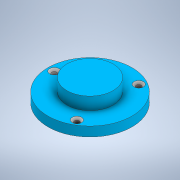
# Autodesk Inventor part: EChem _S200 Cap Base
Saved by Autodesk Inventor 2021 (Build 250183000, 183)
## iProperties
Created: 2020-07-06
Part Number: EChem _S200 Cap Base
Material: Generic
Document SubType Name: Modeling
Designer: jgray
Density: 1 g/cm^3
Appearance: Default
Author: jgray
Autodesk Inventor part; units mm, degrees
ref_plane "YZ Plane" through (0, 0, 0) normal (1, 0, 0) x (0, 1, 0)
ref_plane "XZ Plane" through (0, 0, 0) normal (0, 1, 0) x (-1, 0, 0)
ref_plane "XY Plane" through (0, 0, 0) normal (0, 0, 1) x (1, 0, 0)
sketch "Sketch1" plane through (0, 0, 0) normal (0, 1, 0) x (-1, 0, 0)
  circle A0 centre (0, 0) radius 20
  dimension "d0" = 40
  constraints: 1 centre point, 1 coincident
  measures "d0" diameter of A0
extrude "Extrusion1" add sketch "Sketch1" along normal blind 4.5
sketch "Sketch2" plane through (0, 4.5, 0) normal (0, 1, 0) x (1, 0, 0)
  circle A0 centre (0, 0) radius 11
  dimension "d3" = 22
  constraints: 1 centre point, 1 coincident
  measures "d3" diameter of A0
extrude "Extrusion2" add sketch "Sketch2" along normal blind 6
sketch "Sketch3" plane through (0, 4.5, 0) normal (0, 1, 0) x (1, 0, 0)
  line L0 (0, -21.0157) -> (0, 24.936) construction
  line L1 (-27.3573, 0) -> (21.7209, 0) construction
  circle A0 centre (0, 0) radius 17 construction
  point P0 (-17, 0)
  point P1 (8.5, -14.7224)
  point P2 (8.5, 14.7224)
  dimension "d6" = 34
  dimension "d9" = 360
  constraints: 4 end point, 3 point on line, 1 coincident, 1 horizontal, 1 horizontal alignment, 1 vertical, 6 other
hole "Hole1" at (-17, 4.5, 0) at (8.5, 4.5, 14.7224) at (8.5, 4.5, -14.7224) direction (0, -1, 0) diameter 2.4 end through all countersink diameter 4.4 countersink angle 90 clearance for "Countersunk Flat Head Screw ISO 2009/7046" size "M2" standard "ISO"
body "Solid1"
